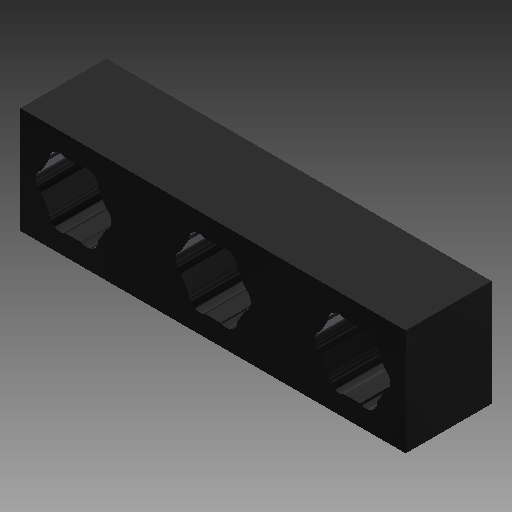
# Autodesk Inventor part: 胴体_サブフレーム_1_2
Saved by Autodesk Inventor 2018 (Build 220112000, 112)
## iProperties
Category: 胴体
Created: 2016-05-07
Part Number: 胴体_サブフレーム_1_2
Material: アセタール樹脂、黒
Document SubType Name: Modeling
Designer: hiroaki
Density: 1.425 g/cm^3
Appearance: 滑らか - 黒
Mass: 2.91382 g
Surface Area: 17.6573 cm^2
Volume: 2.04479 cm^3
Author: hiroaki
Autodesk Inventor part; units mm, degrees
ref_plane "YZ Plane" through (0, 0, 0) normal (1, 0, 0) x (0, 1, 0)
ref_plane "XZ Plane" through (0, 0, 0) normal (0, 1, 0) x (-1, 0, 0)
ref_plane "XY Plane" through (0, 0, 0) normal (0, 0, 1) x (1, 0, 0)
sketch "スケッチ1" plane through (0, 0, 0) normal (0, 0, 1) x (1, 0, 0)
  line L0 (-17.955, -4.955) -> (17.955, -4.955)
  line L1 (17.955, -4.955) -> (17.955, 4.955)
  line L2 (17.955, 4.955) -> (-17.955, 4.955)
  line L3 (-17.955, 4.955) -> (-17.955, -4.955)
  line L4 (-17.955, -4.955) -> (17.955, 4.955) construction
  line L5 (17.955, -4.955) -> (-17.955, 4.955) construction
  circle A0 centre (-13, 0) radius 1.55
  circle A1 centre (0, 0) radius 1.55
  line L6 (0, 0) -> (0, 4.955) construction
  line L7 (-12.5995, 4.955) -> (4.4005, 4.955) construction
  line L8 (-8.5, -4) -> (8.5, -4) construction
  line L9 (-11.2391, -3.05) -> (-14.7609, -3.05)
  line L10 (-14.7609, -3.05) -> (-16.5218, 0)
  line L11 (-16.5218, 0) -> (-14.7609, 3.05)
  line L12 (-14.7609, 3.05) -> (-11.2391, 3.05)
  line L13 (-11.2391, 3.05) -> (-9.4782, 0)
  line L14 (-9.4782, 0) -> (-11.2391, -3.05)
  circle A2 centre (-15.4718, 0) radius 1.05
  circle A3 centre (-14.2359, -2.1407) radius 1.05
  circle A4 centre (-11.7641, -2.1407) radius 1.05
  circle A5 centre (-10.5282, 0) radius 1.05
  circle A6 centre (-11.7641, 2.1407) radius 1.05
  circle A7 centre (-14.2359, 2.1407) radius 1.05
  circle A8 centre (13, 0) radius 1.55
  line L15 (11.2391, -3.05) -> (14.7609, -3.05)
  line L16 (14.7609, -3.05) -> (16.5218, 0)
  line L17 (16.5218, 0) -> (14.7609, 3.05)
  line L18 (14.7609, 3.05) -> (11.2391, 3.05)
  line L19 (11.2391, 3.05) -> (9.4782, 0)
  line L20 (9.4782, 0) -> (11.2391, -3.05)
  circle A9 centre (15.4718, 0) radius 1.05
  circle A10 centre (14.2359, -2.1407) radius 1.05
  circle A11 centre (11.7641, -2.1407) radius 1.05
  circle A12 centre (10.5282, 0) radius 1.05
  circle A13 centre (11.7641, 2.1407) radius 1.05
  circle A14 centre (14.2359, 2.1407) radius 1.05
  circle A15 centre (-13, 0) radius 4.955 construction
  line L21 (1.7609, -3.05) -> (-1.7609, -3.05)
  line L22 (-1.7609, -3.05) -> (-3.5218, 0)
  line L23 (-3.5218, 0) -> (-1.7609, 3.05)
  line L24 (-1.7609, 3.05) -> (1.7609, 3.05)
  line L25 (1.7609, 3.05) -> (3.5218, 0)
  line L26 (3.5218, 0) -> (1.7609, -3.05)
  circle A16 centre (-2.4718, 0) radius 1.05
  circle A17 centre (-1.2359, -2.1407) radius 1.05
  circle A18 centre (1.2359, -2.1407) radius 1.05
  circle A19 centre (2.4718, 0) radius 1.05
  circle A20 centre (1.2359, 2.1407) radius 1.05
  circle A21 centre (-1.2359, 2.1407) radius 1.05
  point P0 (-11.2391, -3.05)
  point P1 (-9.4782, 0)
  point P2 (-11.2391, 3.05)
  point P3 (-14.7609, 3.05)
  point P4 (11.2391, -3.05)
  point P5 (9.4782, 0)
  point P6 (11.2391, 3.05)
  point P7 (14.7609, 3.05)
  point P8 (-1.7609, -3.05)
  point P9 (1.7609, -3.05)
  point P10 (3.5218, 0)
  point P11 (1.7609, 3.05)
  point P12 (-1.7609, 3.05)
  dimension "d19" = 2.1
  dimension "d1" = 3.1
  dimension "d4" = 13
  dimension "d5" = 9.91
  dimension "d20" = 6.1
  dimension "d23" = 360
  dimension "d33" = 360
  constraints: 54 end point, 19 symmetric about line, 9 horizontal alignment, 6 coincident, 6 vertical, 5 horizontal, 5 midpoint, 4 centre point, 2 collinear, 2 parallel, 2 tangent, 1 equal radius, 1 perpendicular, 113 other
  measures "d1" diameter of A0
  measures "d4" distance of point (0, 0) A0.centre
  measures "d5" distance of L2.end L0.start
  measures "d20" distance between parallel lines of L12 L9
extrude "押し出し1" add sketch "スケッチ1" along normal blind 8
equation "\"d4\" = d0"
equation "\"d0\" = 13"
